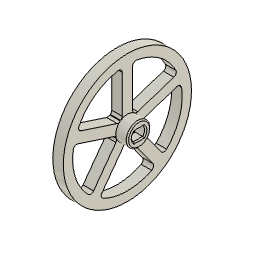
wheel-pololu-tires (Autodesk Fusion 360 design; units mm, degrees)
Autodesk Fusion 360 part; units mm, degrees
sketch "Sketch2" plane through (0, 0, 0) normal (0, 1, 0) x (1, 0, 0)
  line L0 (4.5, 0) -> (4.5, 5)
  line L1 (0, 27.44) -> (4.5, 27.44)
  line L2 (9.5, 0) -> (9.5, 5)
  line L3 (0, 0) -> (4.5, 0)
  line L4 (0, 0) -> (0, 27.44)
  line L5 (4.5, 0) -> (4.5, 27.44)
  line L6 (4.5, 0) -> (9.5, 0)
  line L7 (4.5, 5) -> (9.5, 5)
  dimension "d33" = 27.44
  dimension "d34" = 4.5
  dimension "d36" = 5
  dimension "d37" = 9.5
  constraint horizontal L3
  constraint vertical L4
  constraint horizontal L1
  constraint vertical L5
  constraint horizontal L7
  constraint horizontal L6
  constraint vertical L2
  constraint vertical L0
  measures "d33" distance of L3.start L1.start
  measures "d34" distance of L1.start L1.end
  measures "d36" distance of L2.start L2.end
  measures "d37" distance of L3.start L2.start
revolve "Revolve1" add sketch "Sketch2" angle 360 about axis through (0, 0, 0) along (1, 0, 0)
sketch "Sketch3" plane through (0, 0, 0) normal (1, 0, 0) x (0, 1, 0)
  line L0 (0.8593, -4.9256) -> (11.937, -20.1728)
  line L1 (4.419, -2.3393) -> (15.4967, -17.5865)
  line L2 (4.9501, -0.7048) -> (22.8742, 5.1191)
  line L3 (-0.8593, -4.9256) -> (-11.937, -20.1728)
  line L4 (-3.5904, 3.4798) -> (-21.5145, 9.3037)
  line L5 (-4.9501, -0.7048) -> (-22.8742, 5.1191)
  line L6 (2.2, 4.49) -> (2.2, 23.3365)
  line L7 (3.5904, 3.4798) -> (21.5145, 9.3037)
  line L8 (-2.2, 4.49) -> (-2.2, 23.3365)
  circle A0 centre (0, 0) radius 23.44
  line L9 (-2.0335, 2) -> (2.0304, 2)
  line L10 (-2.0304, -2) -> (2.0304, -2)
  line L11 (-4.419, -2.3393) -> (-15.4967, -17.5865)
  circle A1 centre (0, 0) radius 5
  circle A2 centre (0, 0) radius 2.85
  dimension "d25" = 10
  dimension "d28" = 4
  dimension "d30" = 5.7
  dimension "d31" = 2
  dimension "d32" = 46.88
  constraint horizontal L9
  constraint coincident L9.end A2
  constraint coincident L10.end A2
  constraint coincident L10.start A2
  measures "d25" diameter of A1
  measures "d28" distance of L9 L10
  measures "d30" diameter of A2
  measures "d31" distance of L9 A0.centre
  measures "d32" diameter of A0
extrude "Extrude1" cut sketch "Sketch3" along normal blind 20 contours L0 L3 A0 A1 | L1 L2 A0 A1 | L5 A0 L11 A1 | L4 L8 A0 A1 | L6 L7 A0 A1 | L9 L10 A2
sketch "Sketch4" plane through (0, 0, 0) normal (0, 1, 0) x (1, 0, 0)
  arc A0 (6.25, -2.0955) -> (3.25, -2.0955) centre (4.75, -7.6205) ccw
  arc A1 (3.25, 2.0955) -> (6.25, 2.0955) centre (4.75, 7.6205) ccw
  line L0 (9.5, 2.0955) -> (0, 2.0955)
  line L1 (0, -2.0955) -> (9.5, -2.0955)
extrude "Extrude3" add sketch "Sketch4" along normal mid plane 4.6
sketch "Sketch5" plane through (0, 0, 0) normal (1, 0, 0) x (0, 1, 0)
  circle A0 centre (0, 0) radius 1.5
  circle A1 centre (0, 0) radius 4
extrude "Extrude5" add sketch "Sketch5" along normal blind 1
fillet "Fillet6" radius 0.5 5 edges at (9.5, 0, 2) (9.5, 0, -2) (9.5, -2.85, 0) (9.5, 2.85, 0) (9.5, -1.8081, 4.6616)
fillet "Fillet8" radius 1.5 20 edges at (2.25, -3.5904, 3.4798) (2.25, -21.5145, 9.3037) (2.25, -2.2, 23.3365) (2.25, -2.2, 4.49) (2.25, 2.2, 4.49) (2.25, 3.5904, 3.4798) (2.25, 2.2, 23.3365) (2.25, 21.5145, 9.3037) (2.25, 4.9501, -0.7048) (2.25, 4.419, -2.3393) (2.25, 22.8742, 5.1191) (2.25, 15.4967, -17.5865) (2.25, 11.937, -20.1728) (2.25, 0.8593, -4.9256) (2.25, -0.8593, -4.9256) (2.25, -11.937, -20.1728) (2.25, -4.419, -2.3393) (2.25, -4.9501, -0.7048) (2.25, -15.4967, -17.5865) (2.25, -22.8742, 5.1191)
